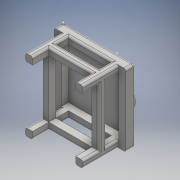
# Autodesk Inventor part: Fantastic6-2
Saved by Autodesk Inventor 2016 (Build 200138000, 138)
## iProperties
Created: 2018-08-06
Part Number: Fantastic6-2
Material: Generic
Document SubType Name: Modeling
Designer: MD
Density: 1 g/cm^3
Appearance: Default
Author: MD
Autodesk Inventor part; units mm, degrees
ref_plane "YZ Plane" through (0, 0, 0) normal (1, 0, 0) x (0, 1, 0)
sketch "Sketch6" plane through (0, 0, 0) normal (0, 1, 0) x (-1, 0, 0)
  line L0 (0, 0) -> (-100, 0)
  line L1 (-100, 0) -> (-100, -100)
  line L2 (-100, -100) -> (0, -100)
  line L3 (0, -100) -> (0, 0)
  dimension "d16" = 100
  dimension "d17" = 100
  constraints: 8 end point, 2 parallel, 1 horizontal, 1 perpendicular
  measures "d16" distance of L2.end L1.end
  measures "d17" distance of L1.end L0.end
extrude "Extrusion5" add sketch "Sketch6" along normal blind 10
sketch "Sketch7" plane through (0, 10, 0) normal (0, 1, 0) x (1, 0, 0)
  line L0 (90, 10) -> (10, 10)
  line L1 (10, 10) -> (10, 90)
  line L2 (10, 90) -> (90, 90)
  line L3 (90, 90) -> (90, 10)
  line L4 (0, 100) -> (0, 0) projected
  line L5 (100, 100) -> (0, 100) projected
  dimension "d20" = 80
  dimension "d21" = 80
  dimension "d22" = 10
  dimension "d23" = 10
  constraints: 8 end point, 2 parallel, 1 horizontal, 1 perpendicular
  measures "d20" distance of L1.end L2.end
  measures "d21" distance of L0.end L1.end
  measures "d22" distance between parallel lines of L4 L1
  measures "d23" distance between parallel lines of L5 L2
extrude "Extrusion6" cut sketch "Sketch7" against normal blind 10
sketch "Sketch8" plane through (0, 10, 0) normal (0, 1, 0) x (1, 0, 0)
  line L0 (100, 0) -> (100, 100) projected
  line L1 (0, 0) -> (100, 0)
  line L2 (100, 0) -> (100, 100)
  line L3 (100, 100) -> (0, 100)
  line L4 (0, 100) -> (0, 0)
  constraints: 8 end point, 2 parallel, 1 horizontal, 1 perpendicular
extrude "Extrusion7" add sketch "Sketch8" along normal blind 3
sketch "Sketch9" plane through (0, 0, 0) normal (0, -1, 0) x (1, 0, 0)
  line L0 (10, -10) -> (10, -90) projected
  line L1 (10, -10) -> (20, -10)
  line L2 (20, -10) -> (20, 0)
  line L3 (20, 0) -> (10, 0)
  line L4 (10, 0) -> (10, -10)
  line L5 (10, -100) -> (20, -100)
  line L6 (20, -100) -> (20, -90)
  line L7 (20, -90) -> (10, -90)
  line L8 (10, -90) -> (10, -100)
  line L9 (80, -10) -> (90, -10)
  line L10 (90, -10) -> (90, 0)
  line L11 (90, 0) -> (80, 0)
  line L12 (80, 0) -> (80, -10)
  line L13 (80, -100) -> (90, -100)
  line L14 (90, -100) -> (90, -90)
  line L15 (90, -90) -> (80, -90)
  line L16 (80, -90) -> (80, -100)
  line L17 (90, -10) -> (90, -90) projected
  point P0 (0, 0)
  dimension "d28" = 10
  dimension "d29" = 10
  dimension "d30" = 10
  dimension "d31" = 10
  dimension "d32" = 10
  dimension "d33" = 10
  dimension "d34" = 10
  dimension "d35" = 10
  dimension "d36" = 0
  dimension "d37" = 0
  constraints: 32 end point, 8 parallel, 4 horizontal, 4 perpendicular
  measures "d28" distance of L3.end L2.end
  measures "d29" distance of L2.end L1.end
  measures "d30" distance of L8.start L7.start
  measures "d31" distance of L7.start L6.start
  measures "d32" distance of L12.start L11.start
  measures "d33" distance of L11.start L10.start
  measures "d34" distance of L16.start L15.start
  measures "d35" distance of L15.start L14.start
  measures "d36" distance between parallel lines of L17 L10
  measures "d37" distance between parallel lines of L17 L14
extrude "Extrusion8" add sketch "Sketch9" along normal blind 50
sketch "Sketch10" plane through (80, 0, -100) normal (-1, 0, 0) x (0, 0, 1)
  line L0 (0, 0) -> (0, -50) projected
  line L1 (0, -17.4889) -> (10, -17.4889)
  line L2 (10, -17.4889) -> (10, -27.4889)
  line L3 (10, -27.4889) -> (0, -27.4889)
  line L4 (0, -27.4889) -> (0, -17.4889)
  line L5 (90, -17.4889) -> (100, -17.4889)
  line L6 (100, -17.4889) -> (100, -27.4889)
  line L7 (100, -27.4889) -> (90, -27.4889)
  line L8 (90, -27.4889) -> (90, -17.4889)
  line L9 (90, 0) -> (90, -50) projected
  point P0 (100, 0)
  dimension "d40" = 10
  dimension "d41" = 10
  dimension "d42" = 10
  dimension "d43" = 10
  dimension "d44" = 0
  constraints: 16 end point, 4 parallel, 2 horizontal, 2 perpendicular, 1 point on line
  measures "d40" distance of L2.end L3.end
  measures "d41" distance of L1.end L2.end
  measures "d42" distance of L6.end L7.end
  measures "d43" distance of L5.end L6.end
  measures "d44" distance between parallel lines of L9 L8
extrude "Extrusion9" add sketch "Sketch10" along normal up to next
sketch "Sketch11" plane through (10, 10, -90) normal (0, 0, 1) x (1, 0, 0)
  line L0 (10, -37.4889) -> (10, -60) projected
  line L1 (10, -37.4889) -> (0, -37.4889)
  line L2 (0, -37.4889) -> (0, -27.4889)
  line L3 (0, -27.4889) -> (10, -27.4889)
  line L4 (10, -27.4889) -> (10, -37.4889)
  line L5 (80, -37.4889) -> (70, -37.4889)
  line L6 (70, -37.4889) -> (70, -27.4889)
  line L7 (70, -27.4889) -> (80, -27.4889)
  line L8 (80, -27.4889) -> (80, -37.4889)
  line L9 (70, -10) -> (70, -27.4889) projected
  point P0 (-10, -10)
  dimension "d47" = 10
  dimension "d48" = 10
  dimension "d49" = 10
  dimension "d50" = 10
  dimension "d51" = 0
  constraints: 16 end point, 4 parallel, 2 horizontal, 2 perpendicular
  measures "d47" distance of L2.end L3.end
  measures "d48" distance of L1.end L2.end
  measures "d49" distance of L7.start L8.start
  measures "d50" distance of L5.end L7.start
  measures "d51" distance between parallel lines of L9 L6
extrude "Extrusion10" add sketch "Sketch11" along normal up to next
sketch "Sketch12" plane through (0, 13, 0) normal (0, 1, 0) x (1, 0, 0)
  point P0 (0, 0)
sketch "Sketch13" plane through (0, 13, 0) normal (0, 1, 0) x (1, 0, 0)
  circle A0 centre (35.0478, 64.2513) radius 15
  circle A1 centre (66.7412, 64.2513) radius 15
  circle A2 centre (50.8214, 36.9315) radius 15
  point P0 (0, 0)
  dimension "d54" = 30
  dimension "d55" = 30
  dimension "d56" = 30
  constraints: 3 centre point
  measures "d54" diameter of A0
  measures "d55" diameter of A1
  measures "d56" diameter of A2
extrude "Extrusion11" add sketch "Sketch13" along normal blind 8
sketch "Sketch14" plane through (50.8214, 21, -36.9315) normal (0, 1, 0) x (1, 0, 0)
  circle A0 centre (0, 0) radius 10
  circle A1 centre (0, 0) radius 5
  circle A2 centre (0, 0) radius 15
  circle A3 centre (-15.7736, 27.3198) radius 15 projected
  circle A4 centre (-15.7736, 27.3198) radius 10
  circle A5 centre (-15.7736, 27.3198) radius 5
  circle A6 centre (-15.7736, 27.3198) radius 15
  circle A7 centre (15.9198, 27.3198) radius 15 projected
  circle A8 centre (15.9198, 27.3198) radius 10
  circle A9 centre (15.9198, 27.3198) radius 5
  circle A10 centre (0, 0) radius 13
  circle A11 centre (-15.7736, 27.3198) radius 13
  circle A12 centre (15.9198, 27.3198) radius 13
  point P0 (-50.8214, -36.9315)
  dimension "d59" = 20
  dimension "d60" = 10
  dimension "d61" = 20
  dimension "d62" = 10
  dimension "d63" = 20
  dimension "d64" = 10
  dimension "d68" = 26
  dimension "d69" = 26
  dimension "d70" = 26
  constraints: 11 centre point, 10 coincident
  measures "d59" diameter of A0
  measures "d60" diameter of A1
  measures "d61" diameter of A4
  measures "d62" diameter of A5
  measures "d63" diameter of A8
  measures "d64" diameter of A9
  measures "d68" diameter of A10
  measures "d69" diameter of A11
  measures "d70" diameter of A12
extrude "Extrusion12" cut sketch "Sketch14" against normal blind 8 contours A1 | A5 | A9 | A10 | A11 | A12
ref_plane "Work Plane1" through (0, 0, -37.5) normal (0, 0, 1) x (1, 0, 0)
sketch "Sketch15" plane through (0, 0, -37.5) normal (0, 0, 1) x (1, 0, 0)
  arc A0 (62.3336, 16.0269) -> (62.3336, 18.8269) centre (62.3336, 17.4269) ccw
  line L0 (62.3336, 16.0269) -> (62.3336, 18.8269)
  point P0 (0, 0)
  dimension "d74" = 2.8
  constraints: 2 end point, 2 point on circle, 1 centre point, 1 vertical
  measures "d74" diameter of A0
revolve "Revolution1" add sketch "Sketch15" angle 360 about axis through (62.3336, 16.0269, -37.5) along (0, 1, 0)
pattern_circular "Circular Pattern1" count 8 over 360 about axis through (50.8214, 21, -36.9315) along (0, -1, 0) of "Revolution1"
ref_plane "Work Plane2" through (0, 0, -64.5) normal (0, 0, 1) x (1, 0, 0)
sketch "Sketch17" plane through (0, 0, -64.5) normal (0, 0, 1) x (1, 0, 0)
  arc A0 (78.2456, 15.5501) -> (78.2456, 18.3501) centre (78.2456, 16.9501) ccw
  line L0 (78.2456, 15.5501) -> (78.2456, 18.3501)
  point P0 (0, 0)
  dimension "d82" = 2.8
  constraints: 2 end point, 2 point on circle, 1 centre point, 1 vertical
  measures "d82" diameter of A0
revolve "Revolution3" add sketch "Sketch17" angle 360 about axis through (78.2456, 15.5501, -64.5) along (0, 1, 0)
pattern_circular "Circular Pattern2" count 8 over 360 about axis through (66.7412, 21, -64.2513) along (0, -1, 0) of "Revolution3"
sketch "Sketch18" plane through (0, 0, -64.5) normal (0, 0, 1) x (1, 0, 0)
  arc A0 (46.5561, 15.4737) -> (46.5561, 18.2737) centre (46.5561, 16.8737) ccw
  line L0 (46.5561, 15.4737) -> (46.5561, 18.2737)
  point P0 (0, 0)
  dimension "d87" = 2.8
  constraints: 2 end point, 2 point on circle, 1 centre point, 1 vertical
  measures "d87" diameter of A0
revolve "Revolution4" add sketch "Sketch18" angle 360 about axis through (46.5561, 15.4737, -64.5) along (0, 1, 0)
pattern_circular "Circular Pattern3" count 8 over 360 about axis through (35.0478, 21, -64.2513) along (0, -1, 0) of "Revolution4"
ref_plane "Work Plane3" through (0, 23.5, 0) normal (0, 1, 0) x (-1, 0, 0)
sketch "Sketch19" plane through (0, 23.5, 0) normal (0, 1, 0) x (-1, 0, 0)
  circle A0 centre (-50.8214, -36.9315) radius 13 projected
  circle A1 centre (-50.8214, -36.9315) radius 15
  circle A2 centre (-50.8214, -36.9315) radius 13
  circle A3 centre (-50.8214, -36.9315) radius 10
  circle A4 centre (-50.8214, -36.9315) radius 5
  circle A5 centre (-66.7412, -64.2513) radius 15 projected
  circle A6 centre (-66.7412, -64.2513) radius 15
  circle A7 centre (-66.7412, -64.2513) radius 13
  circle A8 centre (-66.7412, -64.2513) radius 10
  circle A9 centre (-66.7412, -64.2513) radius 5
  circle A10 centre (-35.0478, -64.2513) radius 15 projected
  circle A11 centre (-35.0478, -64.2513) radius 15
  circle A12 centre (-35.0478, -64.2513) radius 13
  circle A13 centre (-35.0478, -64.2513) radius 10
  circle A14 centre (-35.0478, -64.2513) radius 5
  point P0 (0, 0)
  constraints: 12 centre point, 12 coincident
extrude "Extrusion13" add sketch "Sketch19" along normal blind 8
sketch "Sketch20" plane through (0, 0, -37.5) normal (0, 0, 1) x (1, 0, 0)
  arc A0 (62.3197, 26.2821) -> (62.3197, 29.0821) centre (62.3197, 27.6821) ccw
  line L0 (62.3197, 26.2821) -> (62.3197, 29.0821)
  point P0 (0, 0)
  dimension "d95" = 2.8
  constraints: 2 end point, 2 point on circle, 1 centre point
  measures "d95" diameter of A0
revolve "Revolution5" add sketch "Sketch20" angle 360 about axis through (62.3197, 26.2821, -37.5) along (0, 1, 0)
pattern_circular "Circular Pattern4" count 8 over 360 about axis through (50.8214, 23.5, -36.9315) along (0, 1, 0) of "Revolution5"
sketch "Sketch21" plane through (0, 0, -64.5) normal (0, 0, 1) x (1, 0, 0)
  arc A0 (78.2126, 25.9831) -> (78.2126, 28.7831) centre (78.2126, 27.3831) ccw
  line L0 (78.2126, 25.9831) -> (78.2126, 28.7831)
  point P0 (0, 0)
  dimension "d100" = 2.8
  constraints: 2 end point, 2 point on circle, 1 centre point, 1 vertical
  measures "d100" diameter of A0
revolve "Revolution6" add sketch "Sketch21" angle 360 about axis through (78.2126, 25.9831, -64.5) along (0, 1, 0)
pattern_circular "Circular Pattern5" count 8 over 360 about axis through (66.7412, 23.5, -64.2513) along (0, 1, 0) of "Revolution6"
sketch "Sketch22" plane through (0, 0, -64.5) normal (0, 0, 1) x (1, 0, 0)
  arc A0 (46.5552, 26.1665) -> (46.5552, 28.9665) centre (46.5552, 27.5665) ccw
  line L0 (46.5552, 26.1665) -> (46.5552, 28.9665)
  point P0 (0, 0)
  dimension "d105" = 2.8
  constraints: 2 end point, 2 point on circle, 1 centre point
  measures "d105" diameter of A0
revolve "Revolution7" add sketch "Sketch22" angle 360 about axis through (46.5552, 26.1665, -64.5) along (0, 1, 0)
pattern_circular "Circular Pattern6" count 8 over 360 about axis through (35.0478, 21, -64.2513) along (0, -1, 0) of "Revolution7"
sketch "Sketch24" plane through (0, 13, 0) normal (0, 1, 0) x (1, 0, 0)
  circle A0 centre (50.8214, 36.9315) radius 5 projected
  circle A1 centre (50.8214, 36.9315) radius 4.75
  circle A2 centre (66.7412, 64.2513) radius 5 projected
  circle A3 centre (66.7412, 64.2513) radius 4.75
  circle A4 centre (35.0478, 64.2513) radius 10 projected
  circle A5 centre (35.0478, 64.2513) radius 4.75
  point P0 (0, 0)
  dimension "d113" = 9.5
  dimension "d114" = 9.5
  dimension "d115" = 9.5
  constraints: 3 centre point, 3 coincident
  measures "d113" diameter of A1
  measures "d114" diameter of A3
  measures "d115" diameter of A5
extrude "Extrusion15" add sketch "Sketch24" along normal blind 18.5 contours A1 | A3 | A5
ref_plane "Work Plane4" through (0, 31.5, 0) normal (0, 1, 0) x (-1, 0, 0)
sketch "Sketch25" plane through (0, 31.5, 0) normal (0, 1, 0) x (-1, 0, 0)
  circle A0 centre (-50.8214, -36.9315) radius 5 projected
  circle A1 centre (-50.8214, -36.9315) radius 15
  circle A2 centre (-50.8214, -36.9315) radius 13
  circle A3 centre (-50.8214, -36.9315) radius 10
  circle A4 centre (-50.8214, -36.9315) radius 13 projected
  arc A5 (-48.9299, -24.0699) -> (-53.9213, -24.3066) centre (-50.8214, -36.9315) ccw
  line L0 (-53.9213, -24.3066) -> (-53.206, -27.22)
  line L1 (-49.3664, -27.038) -> (-48.9299, -24.0699)
  circle A6 centre (-50.8214, -36.9315) radius 10
  circle A7 centre (-50.8214, -36.9315) radius 13
  line L2 (-56.7884, -28.9069) -> (-58.5785, -26.4995)
  line L3 (-61.9406, -30.1963) -> (-59.3746, -31.7506)
  circle A8 centre (-50.8214, -36.9315) radius 10
  circle A9 centre (-50.8214, -36.9315) radius 13
  line L4 (-60.715, -35.4766) -> (-63.683, -35.0401)
  line L5 (-63.4464, -40.0315) -> (-60.5329, -39.3161)
  circle A10 centre (-50.8214, -36.9315) radius 10
  circle A11 centre (-50.8214, -36.9315) radius 13
  line L6 (-58.846, -42.8986) -> (-61.2534, -44.6887)
  line L7 (-57.5566, -48.0508) -> (-56.0023, -45.4848)
  circle A12 centre (-50.8214, -36.9315) radius 10
  circle A13 centre (-50.8214, -36.9315) radius 13
  line L8 (-52.2763, -46.8251) -> (-52.7128, -49.7932)
  line L9 (-47.7214, -49.5565) -> (-48.4368, -46.6431)
  circle A14 centre (-50.8214, -36.9315) radius 10
  circle A15 centre (-50.8214, -36.9315) radius 13
  line L10 (-44.8544, -44.9562) -> (-43.0643, -47.3636)
  line L11 (-39.7021, -43.6667) -> (-42.2681, -42.1125)
  circle A16 centre (-50.8214, -36.9315) radius 10
  circle A17 centre (-50.8214, -36.9315) radius 13
  line L12 (-40.9278, -38.3865) -> (-37.9597, -38.823)
  line L13 (-38.1964, -33.8316) -> (-41.1098, -34.5469)
  circle A18 centre (-50.8214, -36.9315) radius 10
  circle A19 centre (-50.8214, -36.9315) radius 13
  line L14 (-42.7967, -30.9645) -> (-40.3893, -29.1744)
  line L15 (-44.0862, -25.8123) -> (-45.6404, -28.3783)
  arc A20 (-58.5785, -26.4995) -> (-61.9406, -30.1963) centre (-50.8214, -36.9315) ccw
  arc A21 (-56.7884, -28.9069) -> (-59.3746, -31.7506) centre (-50.8214, -36.9315) ccw
  arc A22 (-40.3893, -29.1744) -> (-44.0862, -25.8123) centre (-50.8214, -36.9315) ccw
  arc A23 (-42.7967, -30.9645) -> (-45.6404, -28.3783) centre (-50.8214, -36.9315) ccw
  arc A24 (-37.9597, -38.823) -> (-38.1964, -33.8316) centre (-50.8214, -36.9315) ccw
  arc A25 (-63.683, -35.0401) -> (-63.4464, -40.0315) centre (-50.8214, -36.9315) ccw
  arc A26 (-61.2534, -44.6887) -> (-57.5566, -48.0508) centre (-50.8214, -36.9315) ccw
  arc A27 (-60.715, -35.4766) -> (-60.5329, -39.3161) centre (-50.8214, -36.9315) ccw
  arc A28 (-58.846, -42.8986) -> (-56.0023, -45.4848) centre (-50.8214, -36.9315) ccw
  arc A29 (-52.7128, -49.7932) -> (-47.7214, -49.5565) centre (-50.8214, -36.9315) ccw
  arc A30 (-52.7128, -49.7932) -> (-47.7214, -49.5565) centre (-50.8214, -36.9315) ccw
  arc A31 (-52.2763, -46.8251) -> (-48.4368, -46.6431) centre (-50.8214, -36.9315) ccw
  arc A32 (-43.0643, -47.3636) -> (-39.7021, -43.6667) centre (-50.8214, -36.9315) ccw
  arc A33 (-44.8544, -44.9562) -> (-42.2681, -42.1125) centre (-50.8214, -36.9315) ccw
  arc A34 (-37.9597, -38.823) -> (-38.1964, -33.8316) centre (-50.8214, -36.9315) ccw
  arc A35 (-40.9278, -38.3865) -> (-41.1098, -34.5469) centre (-50.8214, -36.9315) ccw
  arc A36 (-40.3893, -29.1744) -> (-44.0862, -25.8123) centre (-50.8214, -36.9315) ccw
  arc A37 (-42.7967, -30.9645) -> (-45.6404, -28.3783) centre (-50.8214, -36.9315) ccw
  point P0 (0, 0)
  dimension "d121" = 360
  constraints: 54 point on circle, 32 end point, 29 coincident, 28 centre point, 107 other
extrude "Extrusion16" add sketch "Sketch25" along normal blind 1 contours A1 | A2 L12 A3 L13 | L14 A3 L15 A2 | A3 | A2 L10 A3 L11 | L1 A3 L0 A2 | A2 L8 A3 L9 | L2 A3 L3 A2 | A2 L6 A3 L7 | L4 A3 L5 A2
sketch "Sketch27" plane through (50.8214, 32.5, -36.9315) normal (0, 1, 0) x (1, 0, 0)
  circle A0 centre (-11.5122, -0.5685) radius 1.75
  point P0 (-50.8214, -36.9315)
  dimension "d125" = 3.5
  constraints: 1 centre point
  measures "d125" diameter of A0
extrude "Extrusion17" add sketch "Sketch27" along normal blind 15
ref_plane "Work Plane5" through (0, 0, -36.5) normal (0, 0, 1) x (1, 0, 0)
sketch "Sketch28" plane through (0, 0, -36.5) normal (0, 0, 1) x (1, 0, 0)
  line L0 (41.0592, 47.5) -> (37.5592, 47.5) projected
  arc A0 (39.3092, 45.1401) -> (39.3092, 49.8599) centre (39.3092, 47.5) ccw
  line L1 (39.3092, 49.8599) -> (39.3092, 45.1401)
  point P0 (0, 0)
  constraints: 2 end point, 2 point on circle, 1 centre point, 1 midpoint, 1 vertical
revolve "Revolution8" add sketch "Sketch28" angle 360 about axis through (39.3092, 49.8599, -36.5) along (0, -1, 0)
fillet "Fillet1" radius 3 38 edges at (100, 6.5, -100) (0, 6.5, -100) (0, 6.5, 0) (100, 6.5, 0) (90, -25, 0) (90, -25, -100) (10, -25, -100) (10, -25, 0) (10, -17.4889, -50) (10, -8.7445, -10) (10, -8.7445, -90) (50, -17.4889, -100) (20, -8.7445, -100) (80, -8.7445, -100) (100, 13, -50) (50, 13, -100) (0, 13, -50) (50, 13, 0) (50, -17.4889, 0) (80, -8.7445, 0) (20, -8.7445, 0) (90, -17.4889, -50) (90, -8.7445, -90) (90, -8.7445, -10) (90, -27.4889, -50) (90, -38.7445, -90) (90, -38.7445, -10) (80, -38.7445, -100) (50, -27.4889, -100) (20, -38.7445, -100) (50, 0, -100) (50, 0, 0) (50, -27.4889, 0) (80, -38.7445, 0) (20, -38.7445, 0) (10, -38.7445, -90) (10, -27.4889, -50) (10, -38.7445, -10)
body "Solid3"
